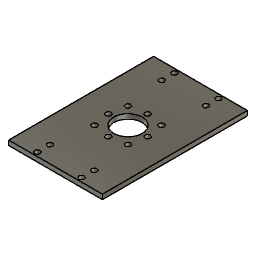
Motor_Mount_LIVE (Autodesk Fusion 360 design; units mm, degrees)
Autodesk Fusion 360 part; units mm, degrees
sketch "Sketch1" plane through (0, 0, 0) normal (0, 0, 1) x (1, 0, 0)
  circle A0 centre (0, 0) radius 29.75
  circle A1 centre (0, 0) radius 12.5
  circle A2 centre (0, 0) radius 15
  circle A3 centre (0, 12.5) radius 1.7
  circle A4 centre (-10.6066, 10.6066) radius 1.7
  circle A5 centre (-10.6066, -10.6066) radius 1.7
  circle A6 centre (-12.5, 0) radius 1.7
  circle A7 centre (10.6066, -10.6066) radius 1.7
  circle A8 centre (0, -12.5) radius 1.7
  circle A9 centre (10.6066, 10.6066) radius 1.7
  circle A10 centre (12.5, 0) radius 1.7
  circle A11 centre (-14, 35.5) radius 1.7
  circle A12 centre (14, 35.5) radius 1.7
  circle A13 centre (14, -35.5) radius 1.7
  circle A14 centre (-14, -35.5) radius 1.7
  line L0 (29.75, 38) -> (29.75, -38)
  line L1 (-29.75, -38) -> (-29.75, 38)
  circle A15 centre (0, 0) radius 9
  line L2 (29.75, 38) -> (29.75, 46)
  line L3 (29.75, 46) -> (-29.75, 46)
  line L4 (-29.75, 46) -> (-29.75, 38)
  circle A16 centre (-14, 43.5) radius 1.7
  circle A17 centre (14, 43.5) radius 1.7
  line L5 (-29.75, -46) -> (29.75, -46)
  line L6 (29.75, -46) -> (29.75, -38)
  line L7 (-29.75, -38) -> (-29.75, -46)
  circle A18 centre (-14, -43.5) radius 1.7
  circle A19 centre (14, -43.5) radius 1.7
  dimension "d1" = 59.5
  dimension "d2" = 25
  dimension "d3" = 30
  dimension "d5" = 3.4
  dimension "d10" = 360
  dimension "d13" = 3.4
  dimension "d14" = 3.4
  dimension "d15" = 3.4
  dimension "d16" = 3.4
  dimension "d17" = 59.5
  dimension "d18" = 76
  dimension "d19" = 18
  dimension "d23" = 8
  dimension "d24" = 3.4
  dimension "d25" = 3.4
  dimension "d27" = 59.5
  dimension "d28" = 8
  dimension "d29" = 3.4
  dimension "d30" = 3.4
  constraint coincident A0.centre A1.centre
  constraint vertical L0
  constraint vertical L1
  constraint vertical L2
  constraint horizontal L3
  constraint vertical L4
  constraint horizontal L5
  constraint vertical L6
  constraint vertical L7
  measures "d1" diameter of A0
  measures "d2" diameter of A1
  measures "d3" diameter of A2
  measures "d5" diameter of A3
  measures "d13" diameter of A11
  measures "d14" diameter of A12
  measures "d15" diameter of A14
  measures "d16" diameter of A13
  measures "d17" distance of L1.end L0.start
  measures "d18" distance of L1.end L1.start
  measures "d19" diameter of A15
  measures "d23" distance of L1.end L3.end
  measures "d24" diameter of A16
  measures "d25" diameter of A17
  measures "d27" distance of L5.end L5.start
  measures "d28" distance of L5.start L1.start
  measures "d29" diameter of A18
  measures "d30" diameter of A19
extrude "Extrude2" add sketch "Sketch1" along normal blind 3 contours A0 | A0 L0 L1 L5 L6 L7 | A0 L0 L1 L2 L3 L4 | A1 A3 A6 A8 A10 | A2 A4 A5 A7 A9
